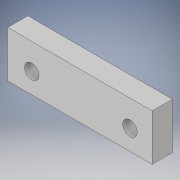
# Autodesk Inventor part: adjustmentHingePlate
Saved by Autodesk Inventor 2017 (Build 210142000, 142)
## iProperties
Created: 2017-04-06
Part Number: adjustmentHingePlate
Material: Generic
Document SubType Name: Modeling
Designer: s4461999
Density: 1 g/cm^3
Appearance: Default
Author: s4461999
Autodesk Inventor part; units mm, degrees
ref_plane "YZ Plane" through (0, 0, 0) normal (1, 0, 0) x (0, 1, 0)
ref_plane "XZ Plane" through (0, 0, 0) normal (0, 1, 0) x (-1, 0, 0)
ref_plane "XY Plane" through (0, 0, 0) normal (0, 0, 1) x (1, 0, 0)
sketch "Sketch1" plane through (0, 0, 0) normal (0, 0, 1) x (1, 0, 0)
  line L0 (0, 0) -> (50, 0)
  line L1 (50, 0) -> (50, 16)
  line L2 (50, 16) -> (0, 16)
  line L3 (0, 16) -> (0, 0)
  dimension "d0" = 50
  dimension "d1" = 16
  constraints: 8 end point, 2 perpendicular, 1 horizontal, 1 parallel
  measures "d0" distance of L0.start L0.end
  measures "d1" distance of L0.end L1.end
extrude "Extrusion1" add sketch "Sketch1" along normal blind 7
sketch "Sketch2" plane through (0, 0, 0) normal (0, 0, -1) x (-1, 0, 0)
  line L0 (0, 0) -> (-50, 0) projected
  point P0 (-8.3598, 7)
  point P1 (-42.3598, 7)
  dimension "d4" = 7
  dimension "d5" = 7
  dimension "d6" = 34
  measures "d4" distance from line of L0 point (-8.36, 7)
  measures "d5" distance from line of L0 point (-42.36, 7)
  measures "d6" distance of point (-42.36, 7) point (-8.36, 7)
hole "Hole1" at (8.3598, 7, 0) at (42.3598, 7, 0) direction (0, 0, 1) diameter 5 end through all
body "Solid1"
